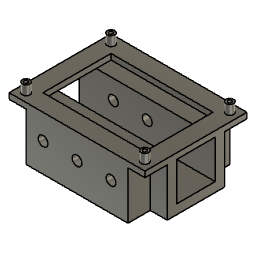
Kinect v1 브라켓 테스트 (Autodesk Fusion 360 design; units mm, degrees)
Autodesk Fusion 360 part; units mm, degrees
note: some values were not read from the file. Set by a fixed rule: which sketch regions a step uses.
sketch "스케치1" plane through (0, 0, 0) normal (0, 0, 1) x (1, 0, 0)
  line L0 (31.5, 22.5) -> (-31.5, 22.5)
  line L1 (-31.5, 22.5) -> (-31.5, -22.5)
  line L2 (-31.5, -22.5) -> (31.5, -22.5)
  line L3 (31.5, -22.5) -> (31.5, 22.5)
  line L4 (31.5, 22.5) -> (-31.5, -22.5) construction
  line L5 (-31.5, 22.5) -> (31.5, -22.5) construction
  circle A0 centre (31.5, 22.5) radius 2
  circle A1 centre (-31.5, 22.5) radius 2
  circle A2 centre (-31.5, -22.5) radius 2
  circle A3 centre (31.5, -22.5) radius 2
  line L6 (36, -27) -> (-36, -27)
  line L7 (-36, -27) -> (-36, 27)
  line L8 (-36, 27) -> (36, 27)
  line L9 (36, 27) -> (36, -27)
  line L10 (36, -27) -> (-36, 27) construction
  line L11 (-36, -27) -> (36, 27) construction
  circle A4 centre (-31.5, 22.5) radius 1
  circle A5 centre (31.5, 22.5) radius 1
  circle A6 centre (31.5, -22.5) radius 1
  circle A7 centre (-31.5, -22.5) radius 1
  line L12 (27, 18) -> (-27, 18)
  line L13 (-27, 18) -> (-27, -18)
  line L14 (-27, -18) -> (27, -18)
  line L15 (27, -18) -> (27, 18)
  line L16 (27, 18) -> (-27, -18) construction
  line L17 (-27, 18) -> (27, -18) construction
  dimension "d1" = 63
  dimension "d2" = 45
  dimension "d3" = 4
  dimension "d4" = 4
  dimension "d5" = 4
  dimension "d6" = 4
  dimension "d7" = 72
  dimension "d8" = 54
  dimension "d9" = 2
  dimension "d10" = 2
  dimension "d11" = 2
  dimension "d12" = 2
  dimension "d13" = 54
  dimension "d14" = 36
  constraint horizontal L0
  constraint perpendicular L0 L1
  constraint parallel L0 L2
  constraint parallel L1 L3
  constraint coincident L4 origin
  constraint coincident L5 origin
  constraint coincident L0.start L3.end
  constraint coincident L0.end L1.start
  constraint coincident L1.end L2.start
  constraint coincident L2.end L3.start
  constraint horizontal L6
  constraint perpendicular L6 L7
  constraint parallel L6 L8
  constraint parallel L7 L9
  constraint coincident L10 origin
  constraint coincident L11 origin
  constraint concentric A1 A4
  constraint concentric A0 A5
  constraint concentric A3 A6
  constraint concentric A2 A7
  constraint horizontal L12
  constraint perpendicular L12 L13
  constraint parallel L12 L14
  constraint parallel L13 L15
  constraint coincident L16 origin
  constraint coincident L17 origin
  measures "d1" distance of L1.end L2.end
  measures "d2" distance of L0.end L1.end
  measures "d3" diameter of A0
  measures "d4" diameter of A1
  measures "d5" diameter of A2
  measures "d6" diameter of A3
  measures "d7" distance of L7.end L8.end
  measures "d8" distance of L6.end L7.end
  measures "d9" diameter of A4
  measures "d10" diameter of A5
  measures "d11" diameter of A6
  measures "d12" diameter of A7
  measures "d13" distance of L13.end L14.end
  measures "d14" distance of L12.end L13.end
extrude "돌출1" add sketch "스케치1" along normal blind 3 contours L0 L1 L2 L3 A0 A1 A2 A3 | L6 L7 L8 L9
extrude "돌출2" add sketch "스케치1" along normal blind 8 contours L0 L1 A1 A4 | L0 L1 A1 A4 | L0 L3 A0 A5 | L0 L3 A0 A5 | L1 L2 A2 A7 | L1 L2 A2 A7 | L2 L3 A3 A6 | L2 L3 A3 A6
sketch "스케치2" plane through (0, 0, 0) normal (1, 0, 0) x (0, 1, 0)
  line L0 (0, 0) -> (0, -25.4)
  line L1 (0, -25.4) -> (15.2, -25.4)
  line L2 (15.2, -25.4) -> (-15.2, -25.4)
  line L3 (-15.2, -25.4) -> (-15.2, 0)
  line L4 (-15.2, 0) -> (15.2, 0)
  line L5 (15.2, 0) -> (15.2, -25.4)
  line L6 (-15.2, -25.4) -> (-10.2, -25.4)
  line L7 (-10.2, -25.4) -> (-10.2, -20.4)
  line L8 (-10.2, -20.4) -> (-15.2, -20.4)
  line L9 (-15.2, -20.4) -> (-15.2, -25.4)
  line L10 (-10.2, -20.4) -> (10.2, -20.4)
  line L11 (10.2, -20.4) -> (10.2, 0)
  line L12 (10.2, 0) -> (-10.2, 0)
  line L13 (-10.2, 0) -> (-10.2, -20.4)
  dimension "d19" = 25.4
  dimension "d20" = 15.2
  dimension "d21" = 30.4
  dimension "d22" = 25.4
  dimension "d23" = 5
  dimension "d24" = 5
  dimension "d25" = 20.4
  constraint coincident L0.start origin
  constraint vertical L0
  constraint perpendicular L0 L1
  constraint horizontal L2
  constraint vertical L3
  constraint horizontal L4
  constraint vertical L5
  constraint horizontal L6
  constraint vertical L7
  constraint horizontal L8
  constraint vertical L9
  constraint horizontal L10
  constraint vertical L11
  constraint horizontal L12
  constraint vertical L13
  measures "d19" distance of L0.start L0.end
  measures "d20" distance of L0.end L1.end
  measures "d21" distance of L1.end L2.end
  measures "d22" distance of L1.end L4.end
  measures "d23" distance of L2.end L6.end
  measures "d24" distance of L2.end L8.end
  measures "d25" distance of L7.end L10.end
extrude "돌출3" add sketch "스케치2" along normal blind 36 contours L0 L1 L2 L4 L5 L10 L11 | L0 L2 L7 L10 | L3 L4 L8 L13 | L2 L3 L6 L7 L8 L9
extrude "돌출4" add 1 faces at (0, -3.4, -23.7333) along direction (-1, 0, 0) blind 36
sketch "스케치3" plane through (0, 15.2, 0) normal (0, 1, 0) x (-1, 0, 0)
  line L0 (27, 0) -> (-27, 0)
  line L1 (-27, 0) -> (-36, 0)
  line L2 (-36, 0) -> (-36, -25.4)
  line L3 (-36, -25.4) -> (36, -25.4)
  line L4 (36, -25.4) -> (36, 0)
  line L5 (36, 0) -> (27, 0)
  line L6 (0, 0) -> (27, 0)
  line L7 (27, 0) -> (-27, 0)
  line L8 (-27, 0) -> (-27, -25.4)
  line L9 (-27, -25.4) -> (27, -25.4)
  line L10 (27, -25.4) -> (27, 0)
  dimension "d30" = 27
  dimension "d31" = 54
  constraint coincident L6.start origin
  constraint parallel L0 L6
  constraint horizontal L7
  constraint vertical L8
  constraint horizontal L9
  constraint vertical L10
  constraint coincident L3 L8.end
  measures "d30" distance of L6.start L0.start
  measures "d31" distance of L0.start L0.end
extrude "돌출5" add sketch "스케치3" along normal blind 11.8 contours L0 L3 L6 L7 L8 L9 L10
sketch "스케치4" plane through (0, -15.2, 0) normal (0, -1, 0) x (1, 0, 0)
  line L0 (-36, -25.4) -> (36, -25.4)
  line L1 (36, -25.4) -> (36, 0)
  line L2 (36, 0) -> (27, 0)
  line L3 (27, 0) -> (-27, 0)
  line L4 (-27, 0) -> (-36, 0)
  line L5 (-36, 0) -> (-36, -25.4)
  line L6 (0, 0) -> (27, 0)
  line L7 (27, 0) -> (-27, 0)
  line L8 (-27, 0) -> (-27, -25.4)
  line L9 (-27, -25.4) -> (27, -25.4)
  line L10 (27, -25.4) -> (27, 0)
  dimension "d34" = 27
  dimension "d35" = 54
  constraint coincident L6.start origin
  constraint parallel L3 L6
  constraint horizontal L7
  constraint vertical L8
  constraint horizontal L9
  constraint vertical L10
  measures "d34" distance of L6.start L2.end
  measures "d35" distance of L2.end L3.end
extrude "돌출6" add sketch "스케치4" along normal blind 11.8 contours L0 L3 L6 L7 L8 L9 L10
sketch "스케치5" plane through (0, 0, -20.4) normal (0, 0, 1) x (-1, 0, 0)
  line L0 (36, 10.2) -> (-36, 10.2)
  line L1 (-36, 10.2) -> (-36, -10.2)
  line L2 (-36, -10.2) -> (36, -10.2)
  line L3 (36, -10.2) -> (36, 10.2)
  line L4 (36, 0) -> (18, 0)
  circle A0 centre (18, 0) radius 2.6
  line L5 (18, 0) -> (0, 0)
  circle A1 centre (0, 0) radius 2.6
  line L6 (0, 0) -> (-18, 0)
  circle A2 centre (-18, 0) radius 2.6
  dimension "d38" = 18
  dimension "d39" = 5.2
  dimension "d40" = 18
  dimension "d41" = 5.2
  dimension "d42" = 18
  dimension "d43" = 5.2
  constraint midpoint L3 L4.start
  constraint perpendicular L3 L4
  constraint coincident L4.end A0.centre
  constraint parallel L4 L5
  constraint coincident L5.end A1.centre
  constraint parallel L5 L6
  constraint coincident L6.end A2.centre
  measures "d38" distance of L4.start L4.end
  measures "d39" diameter of A0
  measures "d40" distance of L4.end L5.end
  measures "d41" diameter of A1
  measures "d42" distance of L5.end L6.end
  measures "d43" diameter of A2
extrude "돌출7" cut sketch "스케치5" against normal blind 12 contours L4 A0 L5 | L4 A0 L5 | L5 A1 L6 | L5 A1 L6 | A2
sketch "스케치6" plane through (0, 10.2, 0) normal (0, -1, 0) x (1, 0, 0)
  line L0 (-36, -20.4) -> (36, -20.4)
  line L1 (36, -20.4) -> (36, 0)
  line L2 (36, 0) -> (27, 0)
  line L3 (27, 0) -> (-27, 0)
  line L4 (-27, 0) -> (-36, 0)
  line L5 (-36, 0) -> (-36, -20.4)
  line L6 (-36, -10.2) -> (-18, -10.2)
  line L7 (-18, -10.2) -> (0, -10.2)
  line L8 (0, -10.2) -> (18, -10.2)
  circle A0 centre (0, -10.2) radius 2.6
  circle A1 centre (18, -10.2) radius 2.6
  circle A2 centre (-18, -10.2) radius 2.6
  dimension "d46" = 5.2
  dimension "d47" = 5.2
  dimension "d48" = 5.2
  constraint midpoint L5 L6.start
  constraint perpendicular L5 L6
  constraint perpendicular L5 L7
  constraint perpendicular L5 L8
  constraint coincident L7.end L8.start
  constraint coincident L8.end A1.centre
  constraint coincident L6.end L7.start
  measures "d46" diameter of A0
  measures "d47" diameter of A1
  measures "d48" diameter of A2
extrude "돌출8" cut sketch "스케치6" against normal blind 16.8 contours L6 L7 A2 | L6 L7 A2 | L7 L8 A0 | L7 L8 A0 | A1
extrude "돌출9" cut sketch "스케치6" along normal blind 53 contours L6 L7 A2 | L6 L7 A2 | L7 L8 A0 | L7 L8 A0 | A1
